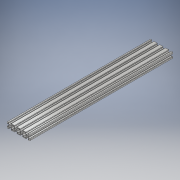
# Autodesk Inventor part: Aluminium Profile 2080 500mm
Saved by Autodesk Inventor 2019 (Build 230136000, 136)
## iProperties
Created: 2020-11-22
Part Number: Aluminium Profile 2080 500mm
Material: Aluminum 6061
Document SubType Name: Modeling
Designer: asus
Density: 2.7 g/cm^3
Appearance: Aluminum - Polished
Author: asus
Autodesk Inventor part; units mm, degrees
ref_plane "YZ Plane" through (0, 0, 0) normal (1, 0, 0) x (0, 1, 0)
ref_plane "XZ Plane" through (0, 0, 0) normal (0, 1, 0) x (-1, 0, 0)
ref_plane "XY Plane" through (0, 0, 0) normal (0, 0, 1) x (1, 0, 0)
sketch "Sketch1" plane through (0, 0, 0) normal (0, 0, 1) x (1, 0, 0)
  line L0 (-33.69, 10) -> (-33.9, 10.21)
  line L1 (-33.9, 10.21) -> (-33.9, 12.8393)
  line L2 (-33.9, 12.8393) -> (-36.5607, 15.5)
  line L3 (-36.5607, 15.5) -> (-38.2, 15.5)
  line L4 (-38.2, 15.5) -> (-38.2, 13.395)
  line L5 (-38.2, 13.395) -> (-38.815, 13.395)
  line L6 (-38.815, 13.395) -> (-40, 14.58)
  line L7 (-40, 14.58) -> (-40, 18.5)
  arc A0 (-38.5, 20) -> (-40, 18.5) centre (-38.5, 18.5) ccw
  line L8 (-38.5, 20) -> (-34.58, 20)
  line L9 (-34.58, 20) -> (-33.395, 18.815)
  line L10 (-33.395, 18.815) -> (-33.395, 18.2)
  line L11 (-33.395, 18.2) -> (-35.5, 18.2)
  line L12 (-35.5, 18.2) -> (-35.5, 16.5607)
  line L13 (-35.5, 16.5607) -> (-32.8393, 13.9)
  line L14 (-32.8393, 13.9) -> (-30.21, 13.9)
  line L15 (-30.21, 13.9) -> (-30, 13.69)
  line L16 (-30, 13.69) -> (-29.79, 13.9)
  line L17 (-29.79, 13.9) -> (-27.1607, 13.9)
  line L18 (-27.1607, 13.9) -> (-24.5, 16.5607)
  line L19 (-24.5, 16.5607) -> (-24.5, 18.2)
  line L20 (-24.5, 18.2) -> (-26.605, 18.2)
  line L21 (-26.605, 18.2) -> (-26.605, 18.815)
  line L22 (-26.605, 18.815) -> (-25.42, 20)
  line L23 (-25.42, 20) -> (-14.58, 20)
  line L24 (-14.58, 20) -> (-13.395, 18.815)
  line L25 (-13.395, 18.815) -> (-13.395, 18.2)
  line L26 (-13.395, 18.2) -> (-15.5, 18.2)
  line L27 (-15.5, 18.2) -> (-15.5, 16.5607)
  line L28 (-15.5, 16.5607) -> (-12.8393, 13.9)
  line L29 (-12.8393, 13.9) -> (-10.21, 13.9)
  line L30 (-10.21, 13.9) -> (-10, 13.69)
  line L31 (-10, 13.69) -> (-9.79, 13.9)
  line L32 (-9.79, 13.9) -> (-7.1607, 13.9)
  line L33 (-7.1607, 13.9) -> (-4.5, 16.5607)
  line L34 (-4.5, 16.5607) -> (-4.5, 18.2)
  line L35 (-4.5, 18.2) -> (-6.605, 18.2)
  line L36 (-6.605, 18.2) -> (-6.605, 18.815)
  line L37 (-6.605, 18.815) -> (-5.42, 20)
  line L38 (-5.42, 20) -> (5.42, 20)
  line L39 (5.42, 20) -> (6.605, 18.815)
  line L40 (6.605, 18.815) -> (6.605, 18.2)
  line L41 (6.605, 18.2) -> (4.5, 18.2)
  line L42 (4.5, 18.2) -> (4.5, 16.5607)
  line L43 (4.5, 16.5607) -> (7.1607, 13.9)
  line L44 (7.1607, 13.9) -> (9.79, 13.9)
  line L45 (9.79, 13.9) -> (10, 13.69)
  line L46 (10, 13.69) -> (10.21, 13.9)
  line L47 (10.21, 13.9) -> (12.8393, 13.9)
  line L48 (12.8393, 13.9) -> (15.5, 16.5607)
  line L49 (15.5, 16.5607) -> (15.5, 18.2)
  line L50 (15.5, 18.2) -> (13.395, 18.2)
  line L51 (13.395, 18.2) -> (13.395, 18.815)
  line L52 (13.395, 18.815) -> (14.58, 20)
  line L53 (14.58, 20) -> (25.42, 20)
  line L54 (25.42, 20) -> (26.605, 18.815)
  line L55 (26.605, 18.815) -> (26.605, 18.2)
  line L56 (26.605, 18.2) -> (24.5, 18.2)
  line L57 (24.5, 18.2) -> (24.5, 16.5607)
  line L58 (24.5, 16.5607) -> (27.1607, 13.9)
  line L59 (27.1607, 13.9) -> (29.79, 13.9)
  line L60 (29.79, 13.9) -> (30, 13.69)
  line L61 (30, 13.69) -> (30.21, 13.9)
  line L62 (30.21, 13.9) -> (32.8393, 13.9)
  line L63 (32.8393, 13.9) -> (35.5, 16.5607)
  line L64 (35.5, 16.5607) -> (35.5, 18.2)
  line L65 (35.5, 18.2) -> (33.395, 18.2)
  line L66 (33.395, 18.2) -> (33.395, 18.815)
  line L67 (33.395, 18.815) -> (34.58, 20)
  line L68 (34.58, 20) -> (38.5, 20)
  arc A1 (40, 18.5) -> (38.5, 20) centre (38.5, 18.5) ccw
  line L69 (40, 18.5) -> (40, 14.58)
  line L70 (40, 14.58) -> (38.815, 13.395)
  line L71 (38.815, 13.395) -> (38.2, 13.395)
  line L72 (38.2, 13.395) -> (38.2, 15.5)
  line L73 (38.2, 15.5) -> (36.5607, 15.5)
  line L74 (36.5607, 15.5) -> (33.9, 12.8393)
  line L75 (33.9, 12.8393) -> (33.9, 10.21)
  line L76 (33.9, 10.21) -> (33.69, 10)
  line L77 (2.7, 16.2393) -> (2.7, 18.2)
  line L78 (2.7, 18.2) -> (-2.7, 18.2)
  line L79 (-2.7, 18.2) -> (-2.7, 16.2393)
  line L80 (-2.7, 16.2393) -> (-6.1, 12.8393)
  line L81 (-6.1, 12.8393) -> (-6.1, 10)
  line L82 (6.1, 10) -> (6.1, 12.8393)
  line L83 (6.1, 12.8393) -> (2.7, 16.2393)
  line L84 (-17.3, 16.2393) -> (-17.3, 18.2)
  line L85 (-17.3, 18.2) -> (-22.7, 18.2)
  line L86 (-22.7, 18.2) -> (-22.7, 16.2393)
  line L87 (-22.7, 16.2393) -> (-26.1, 12.8393)
  line L88 (-26.1, 12.8393) -> (-26.1, 10)
  line L89 (-13.9, 10) -> (-13.9, 12.8393)
  line L90 (-13.9, 12.8393) -> (-17.3, 16.2393)
  line L91 (22.7, 16.2393) -> (22.7, 18.2)
  line L92 (22.7, 18.2) -> (17.3, 18.2)
  line L93 (17.3, 18.2) -> (17.3, 16.2393)
  line L94 (17.3, 16.2393) -> (13.9, 12.8393)
  line L95 (13.9, 12.8393) -> (13.9, 10)
  line L96 (26.1, 10) -> (26.1, 12.8393)
  line L97 (26.1, 12.8393) -> (22.7, 16.2393)
  circle A2 centre (10, 10) radius 2.3
  circle A3 centre (-10, 10) radius 2.3
  circle A4 centre (-30, 10) radius 2.3
  circle A5 centre (30, 10) radius 2.3
  line L98 (-24.5, 1.8) -> (-26.605, 1.8)
  line L99 (-24.5, 3.4393) -> (-24.5, 1.8)
  line L100 (-22.7, 3.7607) -> (-26.1, 7.1607)
  line L101 (-22.7, 1.8) -> (-22.7, 3.7607)
  line L102 (6.1, 7.1607) -> (2.7, 3.7607)
  line L103 (2.7, 1.8) -> (-2.7, 1.8)
  line L104 (-5.42, 0) -> (5.42, 0)
  line L105 (-2.7, 3.7607) -> (-6.1, 7.1607)
  line L106 (-7.1607, 6.1) -> (-4.5, 3.4393)
  line L107 (-2.7, 1.8) -> (-2.7, 3.7607)
  line L108 (-4.5, 3.4393) -> (-4.5, 1.8)
  line L109 (-4.5, 1.8) -> (-6.605, 1.8)
  line L110 (-6.605, 1.8) -> (-6.605, 1.185)
  line L111 (-6.605, 1.185) -> (-5.42, 0)
  line L112 (33.9, 7.1607) -> (33.9, 9.79)
  line L113 (30, 6.31) -> (30.21, 6.1)
  line L114 (33.9, 9.79) -> (33.69, 10)
  line L115 (29.79, 6.1) -> (30, 6.31)
  line L116 (27.1607, 6.1) -> (29.79, 6.1)
  line L117 (30.21, 6.1) -> (32.8393, 6.1)
  line L118 (26.605, 1.185) -> (26.605, 1.8)
  line L119 (25.42, 0) -> (26.605, 1.185)
  line L120 (2.7, 3.7607) -> (2.7, 1.8)
  line L121 (4.5, 1.8) -> (4.5, 3.4393)
  line L122 (6.605, 1.8) -> (4.5, 1.8)
  line L123 (6.605, 1.185) -> (6.605, 1.8)
  line L124 (5.42, 0) -> (6.605, 1.185)
  line L125 (-6.1, 7.1607) -> (-6.1, 10)
  line L126 (4.5, 3.4393) -> (7.1607, 6.1)
  line L127 (-29.79, 6.1) -> (-27.1607, 6.1)
  line L128 (-30, 6.31) -> (-29.79, 6.1)
  line L129 (-30.21, 6.1) -> (-30, 6.31)
  line L130 (-32.8393, 6.1) -> (-30.21, 6.1)
  line L131 (-33.9, 9.79) -> (-33.9, 7.1607)
  line L132 (-33.69, 10) -> (-33.9, 9.79)
  line L133 (-26.1, 7.1607) -> (-26.1, 10)
  line L134 (-27.1607, 6.1) -> (-24.5, 3.4393)
  line L135 (-13.9, 10) -> (-13.9, 7.1607)
  line L136 (-12.8393, 6.1) -> (-10.21, 6.1)
  line L137 (-10.21, 6.1) -> (-10, 6.31)
  line L138 (-10, 6.31) -> (-9.79, 6.1)
  line L139 (-9.79, 6.1) -> (-7.1607, 6.1)
  line L140 (-33.395, 1.185) -> (-33.395, 1.8)
  line L141 (-35.5, 3.4393) -> (-32.8393, 6.1)
  line L142 (-33.395, 1.8) -> (-35.5, 1.8)
  line L143 (-35.5, 1.8) -> (-35.5, 3.4393)
  line L144 (-34.58, 0) -> (-33.395, 1.185)
  line L145 (-33.9, 7.1607) -> (-36.5607, 4.5)
  line L146 (-36.5607, 4.5) -> (-38.2, 4.5)
  line L147 (-38.2, 4.5) -> (-38.2, 6.605)
  line L148 (-38.2, 6.605) -> (-38.815, 6.605)
  line L149 (-38.815, 6.605) -> (-40, 5.42)
  line L150 (-38.5, 0) -> (-34.58, 0)
  arc A6 (-40, 1.5) -> (-38.5, 0) centre (-38.5, 1.5) ccw
  line L151 (-40, 5.42) -> (-40, 1.5)
  line L152 (32.8393, 6.1) -> (35.5, 3.4393)
  line L153 (36.5607, 4.5) -> (33.9, 7.1607)
  line L154 (33.395, 1.8) -> (33.395, 1.185)
  line L155 (38.815, 6.605) -> (38.2, 6.605)
  line L156 (35.5, 1.8) -> (33.395, 1.8)
  line L157 (35.5, 3.4393) -> (35.5, 1.8)
  line L158 (38.2, 4.5) -> (36.5607, 4.5)
  line L159 (38.2, 6.605) -> (38.2, 4.5)
  line L160 (33.395, 1.185) -> (34.58, 0)
  line L161 (40, 5.42) -> (38.815, 6.605)
  line L162 (40, 1.5) -> (40, 5.42)
  arc A7 (38.5, 0) -> (40, 1.5) centre (38.5, 1.5) ccw
  line L163 (34.58, 0) -> (38.5, 0)
  line L164 (13.9, 7.1607) -> (13.9, 10)
  line L165 (26.1, 10) -> (26.1, 7.1607)
  line L166 (12.8393, 6.1) -> (15.5, 3.4393)
  line L167 (17.3, 3.7607) -> (13.9, 7.1607)
  line L168 (15.5, 3.4393) -> (15.5, 1.8)
  line L169 (15.5, 1.8) -> (13.395, 1.8)
  line L170 (17.3, 1.8) -> (17.3, 3.7607)
  line L171 (13.395, 1.8) -> (13.395, 1.185)
  line L172 (22.7, 1.8) -> (17.3, 1.8)
  line L173 (13.395, 1.185) -> (14.58, 0)
  line L174 (14.58, 0) -> (25.42, 0)
  line L175 (22.7, 3.7607) -> (22.7, 1.8)
  line L176 (26.1, 7.1607) -> (22.7, 3.7607)
  line L177 (24.5, 3.4393) -> (27.1607, 6.1)
  line L178 (24.5, 1.8) -> (24.5, 3.4393)
  line L179 (26.605, 1.8) -> (24.5, 1.8)
  line L180 (-26.605, 1.8) -> (-26.605, 1.185)
  line L181 (-13.9, 7.1607) -> (-17.3, 3.7607)
  line L182 (-13.395, 1.8) -> (-15.5, 1.8)
  line L183 (-17.3, 3.7607) -> (-17.3, 1.8)
  line L184 (-15.5, 1.8) -> (-15.5, 3.4393)
  line L185 (-13.395, 1.185) -> (-13.395, 1.8)
  line L186 (-14.58, 0) -> (-13.395, 1.185)
  line L187 (-17.3, 1.8) -> (-22.7, 1.8)
  line L188 (-25.42, 0) -> (-14.58, 0)
  line L189 (-26.605, 1.185) -> (-25.42, 0)
  line L190 (-15.5, 3.4393) -> (-12.8393, 6.1)
  line L191 (7.1607, 6.1) -> (9.79, 6.1)
  line L192 (9.79, 6.1) -> (10, 6.31)
  line L193 (6.1, 10) -> (6.1, 7.1607)
  line L194 (10, 6.31) -> (10.21, 6.1)
  line L195 (10.21, 6.1) -> (12.8393, 6.1)
  constraints: 392 end point, 8 centre point, 8 point on circle
extrude "Extrusion3" add sketch "Sketch1" along normal blind 500
body "Solid3"
